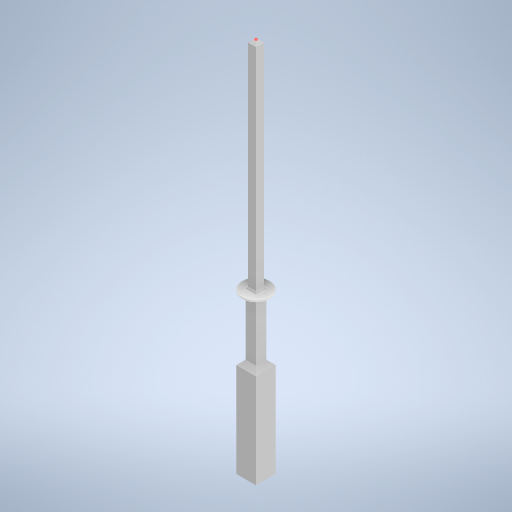
# Autodesk Inventor part: 尖尖
Saved by Autodesk Inventor 2024.2 (Build 282272000, 272)
## iProperties
Created: 2024-06-04
Part Number: 尖尖
Material: 一般
Document SubType Name: Modeling
Designer: sohil
Density: 1 g/cm^3
Appearance: 銀色
Author: sohil
Autodesk Inventor part; units mm, degrees
ref_plane "YZ Plane" through (0, 0, 0) normal (1, 0, 0) x (0, 1, 0)
ref_plane "XZ Plane" through (0, 0, 0) normal (0, 1, 0) x (-1, 0, 0)
ref_plane "XY Plane" through (0, 0, 0) normal (0, 0, 1) x (1, 0, 0)
sketch "草圖1" plane through (0, 0, 0) normal (0, 1, 0) x (-1, 0, 0)
  line L0 (0, 0) -> (-10, 0)
  line L1 (-10, 0) -> (-10, -10)
  line L2 (-10, -10) -> (0, -10)
  line L3 (0, -10) -> (0, 0)
  dimension "d0" = 10
  dimension "d1" = 10
  constraints: 8 end point, 2 parallel, 1 horizontal, 1 perpendicular
  measures "d0" distance of L2.end L1.end
  measures "d1" distance of L1.end L0.end
extrude "擠出1" add sketch "草圖1" along normal blind 50
chamfer "倒角1" distance 2.4 angle 45 4 edges at (5, 50, 0) (10, 50, -5) (5, 50, -10) (0, 50, -5)
sketch "草圖2" plane through (0, 50, 0) normal (0, 1, 0) x (1, 0, 0)
  line L0 (2.4, 2.4) -> (2.4, 7.6) projected
  line L1 (7.6, 2.4) -> (2.4, 2.4) projected
  line L2 (2.4, 7.6) -> (7.6, 7.6)
  line L3 (7.6, 7.6) -> (7.6, 2.4)
  line L4 (7.6, 2.4) -> (2.4, 2.4)
  line L5 (2.4, 2.4) -> (2.4, 7.6)
  point P0 (0, 0)
  constraints: 8 end point, 2 parallel, 1 horizontal, 1 perpendicular
extrude "擠出2" add sketch "草圖2" along normal blind 30
sketch "草圖3" plane through (0, 80, 0) normal (0, 1, 0) x (1, 0, 0)
  line L0 (2.4, 7.6) -> (7.6, 7.6)
  line L1 (7.6, 7.6) -> (7.6, 2.4)
  line L2 (7.6, 2.4) -> (2.4, 2.4)
  line L3 (2.4, 2.4) -> (2.4, 7.6)
  circle A0 centre (5, 5) radius 7.0711
  line L4 (7, 7) -> (3, 7)
  line L5 (3, 7) -> (3, 3)
  line L6 (3, 3) -> (7, 3)
  line L7 (7, 3) -> (7, 7)
  line L8 (7, 7) -> (3, 3) construction
  line L9 (3, 7) -> (7, 3) construction
  point P0 (0, 0)
  point P1 (10, 10)
  dimension "d31" = 4
  dimension "d32" = 4
  constraints: 20 end point, 4 parallel, 3 perpendicular, 2 midpoint, 1 horizontal, 3 other
  measures "d31" distance of L4.start L4.end
  measures "d32" distance of L5.end L4.end
extrude "擠出3" add sketch "草圖3" along normal blind 110 contours L7 L6 L5 L4
extrude "擠出5" add sketch "草圖3" along normal blind 1 contours A0
fillet "圓角1" radius 0.2 2 edges at (-2.0711, 80, -5) (-2.0711, 81, -5)
chamfer "倒角7" distance 1.25 angle 45 4 edges at (5, 190, -7) (7, 190, -5) (5, 190, -3) (3, 190, -5)
extrude "擠出6" add sketch "草圖3" along normal blind 2 contours L0 L1 L2 L3 | L7 L6 L5 L4
chamfer "倒角8" distance 1 angle 30 1 edges at (5, 82, -7.6) measured on face at (5.8667, 81.3333, -7.6)
chamfer "倒角9" distance 1 angle 30 1 edges at (2.4, 82, -4.7116) measured on face at (2.4, 81.3333, -5.6744)
chamfer "倒角10" distance 1 angle 30 1 edges at (5.2884, 82, -2.4) measured on face at (4.3256, 81.3333, -2.4)
chamfer "倒角11" distance 1 angle 30 1 edges at (7.6, 82, -5) measured on face at (7.6, 81.3333, -5.6744)
sketch "草圖7" plane through (0, 190, 0) normal (0, 1, 0) x (1, 0, 0)
  line L0 (5.75, 5.75) -> (5.75, 4.25) projected
  circle A0 centre (5, 5) radius 0.725
  line L1 (5.75, 5) -> (4.25, 5)
  point P0 (0, 0)
  point P1 (5.725, 5)
  point P2 (4.275, 5)
  dimension "d54" = 1.45
  constraints: 2 end point, 1 centre point, 1 midpoint, 1 perpendicular
  measures "d54" diameter of A0
revolve "迴轉2" add sketch "草圖7" angle 180 about axis through (5.75, 190, -5) along (-1, 0, 0) picked at (4.7654, 4.9422) contours A0 L1
sketch "草圖9" plane through (0, 190, 0) normal (0, 1, 0) x (1, 0, 0)
  circle A0 centre (5, 5) radius 0.725
  circle A1 centre (5, 5) radius 0.75
  point P0 (0, 0)
  constraints: 2 centre point, 2 coincident
extrude "擠出8" add sketch "草圖9" along normal blind 0.1 contours A0 | A1
